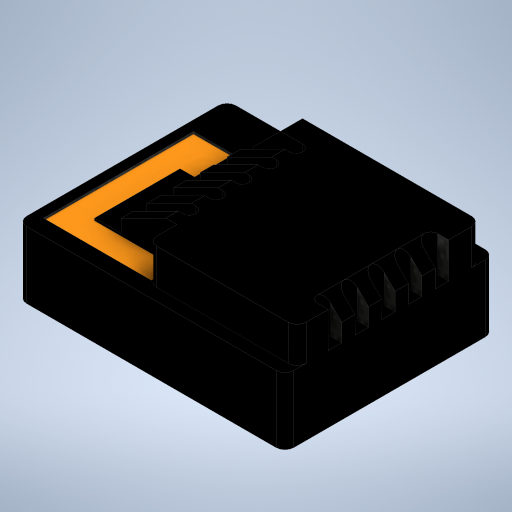
# Autodesk Inventor part: Motor-controlling
Saved by Autodesk Inventor 2023 (Build 270158000, 158)
## iProperties
Created: 2023-01-12
Part Number: Motor-controlling
Material: Steel
Document SubType Name: Modeling
Designer: t205b
Density: 7.85 g/cm^3
Appearance: Plate
Mass: 424.821 g
Surface Area: 109.929 cm^2
Volume: 54.1173 cm^3
Author: t205b
Autodesk Inventor part; units mm, degrees
ref_plane "YZ Plane" through (0, 0, 0) normal (1, 0, 0) x (0, 1, 0)
ref_plane "XZ Plane" through (0, 0, 0) normal (0, 1, 0) x (-1, 0, 0)
ref_plane "XY Plane" through (0, 0, 0) normal (0, 0, 1) x (1, 0, 0)
sketch "Sketch1" plane through (0, 0, 0) normal (0, 1, 0) x (-1, 0, 0)
  line L0 (25.931, 23.0273) -> (-34.069, 23.0273)
  line L1 (-34.069, 23.0273) -> (-34.069, -23.9727)
  line L2 (-34.069, -23.9727) -> (25.931, -23.9727)
  line L3 (25.931, -23.9727) -> (25.931, 23.0273)
  point P0 (0, 0)
  dimension "d0" = 47
  dimension "d1" = 60
  constraints: 8 end point, 2 parallel, 1 horizontal, 1 perpendicular
  measures "d0" distance of L2.end L0.start
  measures "d1" distance of L1.end L2.end
extrude "Extrusion1" add sketch "Sketch1" along normal blind 15
fillet "Fillet1" radius 2 4 edges at (34.069, 7.5, 23.0273) (34.069, 7.5, -23.9727) (-25.931, 7.5, 23.0273) (-25.931, 7.5, -23.9727)
sketch "Sketch2" plane through (0, 15, 0) normal (0, 1, 0) x (1, 0, 0)
  arc A0 (34.069, 21.9727) -> (32.069, 23.9727) centre (32.069, 21.9727) ccw projected
  line L0 (34.069, -20.2773) -> (0.569, -20.2773)
  line L1 (0.569, -20.2773) -> (0.569, -13.7773)
  line L2 (0.569, -13.7773) -> (-11.931, -13.7773)
  line L3 (-11.931, -13.7773) -> (-11.931, 20.9227)
  line L4 (34.069, -20.2773) -> (34.069, 20.9227)
  line L5 (34.069, -21.0273) -> (34.069, 21.9727) projected
  line L6 (-11.931, 20.9227) -> (34.069, 20.9227)
  line L7 (-23.931, -23.0273) -> (32.069, -23.0273) projected
  point P0 (0, 0)
  dimension "d5" = 33.5
  dimension "d6" = 41.2
  dimension "d7" = 2.75
  dimension "d8" = 6.5
  dimension "d9" = 46
  constraints: 12 end point, 3 perpendicular, 1 horizontal, 1 point on line, 1 vertical
  measures "d5" distance of L0.start L0.end
  measures "d6" distance between parallel lines of L0 L6
  measures "d7" distance between parallel lines of L7 L0
  measures "d8" distance of L0.end L1.end
  measures "d9" distance between parallel lines of L3 L4
extrude "Extrusion2" add sketch "Sketch2" along normal blind 8
fillet "Fillet2" radius 2 3 edges at (34.069, 19, -20.9227) (34.069, 19, 20.2773) (0.569, 19, 20.2773)
sketch "Sketch3" plane through (-11.931, 15, 13.7773) normal (0, 0, 1) x (1, 0, 0)
  line L0 (44, 8) -> (0, 8) projected
  line L1 (10, 8) -> (0, 8)
  line L2 (0, 0) -> (0, 8) projected
  line L3 (10, 8) -> (0, 3)
  line L4 (0, 0) -> (0, 8) projected
  line L5 (-12, 0) -> (44, 0) projected
  point P0 (11.931, -15)
  dimension "d13" = 10
  dimension "d14" = 3
  constraints: 4 end point, 2 point on line, 1 collinear
  measures "d13" distance from line of L1.start L2
  measures "d14" distance from line of L3.end L5
extrude "Extrusion3" cut sketch "Sketch3" against normal blind 27
sketch "Sketch4" plane through (-11.931, 15, -20.9227) normal (0, 0, -1) x (-1, 0, 0)
  line L0 (-44, 8) -> (0, 8) projected
  line L1 (-6, 8) -> (0, 2)
  line L2 (0, 0) -> (0, 8) projected
  point P0 (-11.931, -15)
  dimension "d17" = 6
  dimension "d18" = 6
  constraints: 2 end point, 2 point on line
  measures "d17" distance from line of L2 L1.start
  measures "d18" distance from line of L0 L1.end
extrude "Extrusion4" cut sketch "Sketch4" against normal blind 5
sketch "Sketch5" plane through (0, 23, 0) normal (0, 1, 0) x (1, 0, 0)
  line L0 (-11.931, -13.7773) -> (-11.931, 13.2227) projected
  line L1 (-11.931, -11.0273) -> (-0.931, -11.0273)
  line L2 (-11.931, -8.0273) -> (-0.931, -8.0273)
  arc A0 (-0.931, -11.0273) -> (-0.931, -8.0273) centre (-0.931, -9.5273) ccw
  line L3 (-1.931, -13.7773) -> (-11.931, -13.7773) projected
  line L4 (-11.931, -2.0273) -> (-0.931, -2.0273)
  arc A1 (-0.931, -5.0273) -> (-0.931, -2.0273) centre (-0.931, -3.5273) ccw
  line L5 (-11.931, -5.0273) -> (-0.931, -5.0273)
  line L6 (-11.931, 3.9727) -> (-0.931, 3.9727)
  arc A2 (-0.931, 0.9727) -> (-0.931, 3.9727) centre (-0.931, 2.4727) ccw
  line L7 (-11.931, 0.9727) -> (-0.931, 0.9727)
  line L8 (-11.931, 9.9727) -> (-0.931, 9.9727)
  arc A3 (-0.931, 6.9727) -> (-0.931, 9.9727) centre (-0.931, 8.4727) ccw
  line L9 (-11.931, 6.9727) -> (-0.931, 6.9727)
  line L10 (-11.931, 15.9727) -> (-0.931, 15.9727)
  arc A4 (-0.931, 12.9727) -> (-0.931, 15.9727) centre (-0.931, 14.4727) ccw
  line L11 (-11.931, 12.9727) -> (-0.931, 12.9727)
  line L12 (-11.931, 15.9227) -> (-11.931, 13.2227) projected
  line L13 (-11.931, 15.9727) -> (-11.931, 12.9727)
  point P0 (0, 0)
  dimension "d21" = 3
  dimension "d22" = 1.5
  dimension "d23" = 2.75
  dimension "d24" = 11
  dimension "d27" = 6
  constraints: 22 end point, 10 point on circle, 5 centre point, 2 horizontal, 2 point on line, 1 collinear, 1 vertical, 32 other
  measures "d21" distance between parallel lines of L1 L2
  measures "d22" radius of A0
  measures "d23" distance between parallel lines of L3 L1
  measures "d24" distance of L1.start L1.end
  measures "d27" distance of L2.start L4.start
extrude "Extrusion5" cut sketch "Sketch5" against normal blind 8
sketch "Sketch6" plane through (0, 23, 0) normal (0, 1, 0) x (1, 0, 0)
  line L0 (34.069, -18.2773) -> (34.069, 18.9227) projected
  line L1 (34.069, -13.2773) -> (31.569, -13.2773)
  line L2 (34.069, -10.2773) -> (31.569, -10.2773)
  arc A0 (31.569, -10.2773) -> (31.569, -13.2773) centre (31.569, -11.7773) ccw
  line L3 (2.569, -20.2773) -> (32.069, -20.2773) projected
  line L4 (34.069, -4.2773) -> (31.569, -4.2773)
  arc A1 (31.569, -4.2773) -> (31.569, -7.2773) centre (31.569, -5.7773) ccw
  line L5 (34.069, -7.2773) -> (31.569, -7.2773)
  line L6 (34.069, 1.7227) -> (31.569, 1.7227)
  arc A2 (31.569, 1.7227) -> (31.569, -1.2773) centre (31.569, 0.2227) ccw
  line L7 (34.069, -1.2773) -> (31.569, -1.2773)
  line L8 (34.069, 7.7227) -> (31.569, 7.7227)
  arc A3 (31.569, 7.7227) -> (31.569, 4.7227) centre (31.569, 6.2227) ccw
  line L9 (34.069, 4.7227) -> (31.569, 4.7227)
  line L10 (34.069, 13.7227) -> (31.569, 13.7227)
  arc A4 (31.569, 13.7227) -> (31.569, 10.7227) centre (31.569, 12.2227) ccw
  line L11 (34.069, 10.7227) -> (31.569, 10.7227)
  point P0 (0, 0)
  dimension "d35" = 1.5
  dimension "d36" = 3
  dimension "d37" = 2.5
  dimension "d38" = 7
  dimension "d41" = 6
  constraints: 20 end point, 10 point on circle, 5 centre point, 2 horizontal, 2 point on line, 1 vertical, 32 other
  measures "d35" radius of A0
  measures "d36" distance between parallel lines of L1 L2
  measures "d37" distance of L1.start L1.end
  measures "d38" distance between parallel lines of L3 L1
  measures "d41" distance of L2.start L4.start
extrude "Extrusion6" cut sketch "Sketch6" against normal blind 8
sketch "Sketch7" plane through (31.569, 23, 10.2773) normal (0, 0, 1) x (1, 0, 0)
  line L0 (-1.5, 0) -> (0, 0) projected
  line L1 (2.5, -8) -> (2.5, 0) projected
  line L2 (2.5, 0) -> (0, 0) projected
  line L3 (2.5, -4) -> (-1.5, 0)
  point P0 (-31.569, -23)
  dimension "d52" = 4
  dimension "d53" = 4
  constraints: 2 end point, 1 midpoint, 1 point on line
  measures "d52" distance from line of L2 L3.start
  measures "d53" distance from line of L1 L3.end
extrude "Extrusion7" cut sketch "Sketch7" against normal blind 22.5
extrude "Extrusion8" cut sketch "Sketch7" along normal blind 1.5
sketch "Sketch9" plane through (0, 15, 0) normal (0, 1, 0) x (1, 0, 0)
  line L0 (-14.681, 14.1727) -> (-23.681, 14.1727)
  line L1 (-23.681, 14.1727) -> (-23.681, -19.5273)
  line L2 (-23.681, -19.5273) -> (0.569, -19.5273)
  line L3 (0.569, -19.5273) -> (0.569, -13.7773)
  line L4 (0.569, -13.7773) -> (-17.931, -13.7773)
  line L5 (-17.931, -13.7773) -> (-17.931, 5.4227)
  line L6 (-17.931, 5.4227) -> (-14.681, 5.4227)
  line L7 (-14.681, 5.4227) -> (-14.681, 14.1727)
  line L8 (-25.931, 21.9727) -> (-25.931, -21.0273) projected
  line L9 (-23.931, -23.0273) -> (32.069, -23.0273) projected
  point P0 (0, 0)
  dimension "d58" = 9
  dimension "d59" = 5.75
  dimension "d60" = 24.25
  dimension "d61" = 33.7
  dimension "d62" = 8.75
  dimension "d63" = 2.25
  dimension "d64" = 3.5
  dimension "d65" = 5.75
  constraints: 16 end point, 4 perpendicular, 3 vertical, 1 horizontal
  measures "d58" distance between parallel lines of L7 L1
  measures "d59" distance between parallel lines of L5 L1
  measures "d60" distance between parallel lines of L1 L3
  measures "d61" distance between parallel lines of L2 L0
  measures "d62" distance of L6.end L0.start
  measures "d63" distance between parallel lines of L1 L8
  measures "d64" distance between parallel lines of L9 L2
  measures "d65" distance between parallel lines of L2 L4
extrude "Extrusion9" cut sketch "Sketch9" against normal blind 0.5
body "Solid1"
